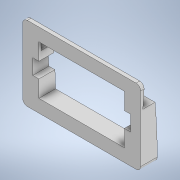
# Autodesk Inventor part: electricalCoverGasket02
Saved by Autodesk Inventor 2021.1 (Build 251245000, 245)
## iProperties
Created: 2020-08-29
Part Number: electricalCoverGasket02
Material: Generic
Document SubType Name: Modeling
Designer: robst
Density: 1 g/cm^3
Appearance: Default
Author: robst
Autodesk Inventor part; units mm, degrees
ref_plane "YZ Plane" through (0, 0, 0) normal (1, 0, 0) x (0, 1, 0)
ref_plane "XZ Plane" through (0, 0, 0) normal (0, 1, 0) x (-1, 0, 0)
sketch "Sketch1" plane through (0, 0, 0) normal (1, 0, 0) x (0, 1, 0)
  line L0 (0, 0) -> (0, 12.7)
  line L1 (0, 0) -> (-101.6, 0) construction
  arc A0 (-101.6, 0) -> (0, 0) centre (-50.8, 556.4861) ccw
  line L2 (-50.8, -2.3139) -> (-50.8, 0) construction
  line L3 (0, 12.7) -> (101.6, 12.7) construction
  arc A1 (0, 12.7) -> (101.6, 12.7) centre (50.8, 569.1861) ccw
  line L4 (22.2779, 14.9245) -> (-55.1921, 14.9245)
  line L5 (-55.1921, 14.9245) -> (-55.1921, -2.2966)
  line L6 (22.2779, 14.9245) -> (22.2779, 11.1145)
  dimension "d5" = 558.8
  dimension "d6" = 101.6
  dimension "d7" = 558.8
  dimension "d24" = 12.7
  dimension "d26" = 77.47
  dimension "d28" = 55.1921
  dimension "d29" = 3.81
  constraints: 14 end point, 7 point on circle, 3 horizontal, 2 centre point, 2 perpendicular, 1 midpoint, 1 vertical
  measures "d5" radius of A0
  measures "d6" distance of L0.end L3.end
  measures "d7" radius of A1
  measures "d24" distance of L0.start L0.end
  measures "d26" distance of L4.start L4.end
  measures "d28" distance between parallel lines of L0 L5
  measures "d29" distance of L4.start L6.end
extrude "Extrusion3" add sketch "Sketch1" along normal mid plane 122.428
sketch "Sketch5" plane through (0, 0, 0) normal (0, 0, 1) x (1, 0, 0)
  line L0 (-61.214, 22.2779) -> (61.214, 22.2779) projected
  line L1 (-61.214, 0) -> (61.214, 0) projected
  line L2 (61.214, 0) -> (61.214, 22.2779)
  line L3 (-61.214, 22.2779) -> (-61.214, 0)
  line L4 (61.214, 14.6579) -> (-61.214, 14.6579) construction
  line L5 (-61.214, -55.1921) -> (-61.214, 22.2779) construction
  line L6 (21.5694, 10.8479) -> (21.5694, 17.5664)
  line L7 (21.5694, 17.5664) -> (24.1259, 17.5664)
  line L8 (24.1259, 17.5664) -> (24.1259, 18.4679)
  line L9 (24.1259, 18.4679) -> (18.0002, 18.4679)
  line L10 (18.0002, 18.4679) -> (18.0002, 17.5664)
  line L11 (18.0002, 17.5664) -> (20.5567, 17.5664)
  line L12 (20.5567, 17.5664) -> (20.5567, 10.8479)
  line L13 (20.5567, 10.8479) -> (21.5694, 10.8479)
  spline S0 degree 2 poles (11.8314, 17.5972) (11.3991, 17.0909) (10.9175, 15.6089) (10.9175, 14.6579) knots 0 0 0 1 2 2 2
  spline S1 degree 2 poles (10.9175, 14.6579) (10.9175, 13.7317) (11.3868, 12.2311) (11.8314, 11.7248) knots 0 0 0 1 2 2 2
  spline S2 degree 2 poles (11.8314, 11.7248) (12.3007, 11.1937) (13.5419, 10.6874) (14.289, 10.6874) knots 0 0 0 1 2 2 2
  spline S3 degree 2 poles (14.289, 10.6874) (15.0609, 10.6874) (16.2959, 11.2122) (16.7467, 11.7248) knots 0 0 0 1 2 2 2
  spline S4 degree 2 poles (16.7467, 11.7248) (17.1851, 12.2311) (17.6544, 13.7193) (17.6544, 14.6579) knots 0 0 0 1 2 2 2
  spline S5 degree 2 poles (17.6544, 14.6579) (17.6544, 15.615) (17.179, 17.0724) (16.7405, 17.5972) knots 0 0 0 1 2 2 2
  spline S6 degree 2 poles (16.7405, 17.5972) (16.2959, 18.1036) (15.0547, 18.6285) (14.289, 18.6285) knots 0 0 0 1 2 2 2
  spline S7 degree 2 poles (14.289, 18.6285) (13.511, 18.6285) (12.2636, 18.0851) (11.8314, 17.5972) knots 0 0 0 1 2 2 2
  spline S8 degree 2 poles (11.9734, 14.6579) (11.9734, 15.4113) (12.3007, 16.5784) (12.5971, 16.9612) knots 0 0 0 1 2 2 2
  spline S9 degree 2 poles (12.5971, 16.9612) (12.8997, 17.3564) (13.7518, 17.7516) (14.2829, 17.7516) knots 0 0 0 1 2 2 2
  spline S10 degree 2 poles (14.2829, 17.7516) (14.8324, 17.7516) (15.6599, 17.3688) (15.9748, 16.9612) knots 0 0 0 1 2 2 2
  spline S11 degree 2 poles (15.9748, 16.9612) (16.2774, 16.5722) (16.5985, 15.3989) (16.5985, 14.6579) knots 0 0 0 1 2 2 2
  spline S12 degree 2 poles (16.5985, 14.6579) (16.5985, 13.1574) (15.3388, 11.5642) (14.2829, 11.5642) knots 0 0 0 1 2 2 2
  spline S13 degree 2 poles (14.2829, 11.5642) (13.2269, 11.5642) (11.9734, 13.1574) (11.9734, 14.6579) knots 0 0 0 1 2 2 2
  spline S14 degree 2 poles (4.9894, 16.1708) (4.9894, 15.6768) (5.3414, 14.7876) (5.6563, 14.4788) knots 0 0 0 1 2 2 2
  spline S15 degree 2 poles (5.6563, 14.4788) (6.0515, 14.0898) (7.1198, 13.6884) (7.9349, 13.6884) knots 0 0 0 1 2 2 2
  line L14 (7.9349, 13.6884) -> (8.7933, 13.6884)
  line L15 (8.7933, 13.6884) -> (8.7933, 10.8479)
  line L16 (8.7933, 10.8479) -> (9.806, 10.8479)
  line L17 (9.806, 10.8479) -> (9.806, 18.4679)
  line L18 (9.806, 18.4679) -> (7.8917, 18.4679)
  spline S16 degree 2 poles (7.8917, 18.4679) (7.2124, 18.4679) (6.2615, 18.2456) (5.8972, 17.9924) knots 0 0 0 1 2 2 2
  spline S17 degree 2 poles (5.8972, 17.9924) (5.4711, 17.7022) (4.9894, 16.8068) (4.9894, 16.1708) knots 0 0 0 1 2 2 2
  spline S18 degree 2 poles (6.0454, 16.1399) (6.0454, 16.5351) (6.3171, 17.1156) (6.5949, 17.3008) knots 0 0 0 1 2 2 2
  spline S19 degree 2 poles (6.5949, 17.3008) (6.8358, 17.4614) (7.478, 17.5911) (7.9535, 17.5911) knots 0 0 0 1 2 2 2
  line L19 (7.9535, 17.5911) -> (8.7933, 17.5911)
  line L20 (8.7933, 17.5911) -> (8.7933, 14.5529)
  line L21 (8.7933, 14.5529) -> (8.1017, 14.5529)
  spline S20 degree 2 poles (8.1017, 14.5529) (7.4841, 14.5529) (6.7246, 14.7505) (6.4776, 15.0099) knots 0 0 0 1 2 2 2
  spline S21 degree 2 poles (6.4776, 15.0099) (6.2491, 15.2384) (6.0454, 15.7756) (6.0454, 16.1399) knots 0 0 0 1 2 2 2
  line L22 (1.0745, 18.8075) -> (4.057, 9.193)
  line L23 (4.057, 9.193) -> (4.9215, 9.193)
  line L24 (4.9215, 9.193) -> (1.9513, 18.8075)
  line L25 (1.9513, 18.8075) -> (1.0745, 18.8075)
  spline S22 degree 2 poles (-5.15, 13.1883) (-5.15, 12.6202) (-4.7177, 11.7495) (-4.3596, 11.4654) knots 0 0 0 1 2 2 2
  spline S23 degree 2 poles (-4.3596, 11.4654) (-3.9273, 11.132) (-2.9455, 10.8479) (-2.1674, 10.8479) knots 0 0 0 1 2 2 2
  line L26 (-2.1674, 10.8479) -> (0.0185, 10.8479)
  line L27 (0.0185, 10.8479) -> (0.0185, 18.4679)
  line L28 (0.0185, 18.4679) -> (-2.0007, 18.4679)
  spline S24 degree 2 poles (-2.0007, 18.4679) (-2.8158, 18.4679) (-3.6309, 18.3629) (-4.0014, 18.1592) knots 0 0 0 1 2 2 2
  spline S25 degree 2 poles (-4.0014, 18.1592) (-4.4152, 17.943) (-4.7918, 17.2329) (-4.7918, 16.7513) knots 0 0 0 1 2 2 2
  spline S26 degree 2 poles (-4.7918, 16.7513) (-4.7918, 16.214) (-4.2237, 15.3619) (-3.7235, 15.121) knots 0 0 0 1 2 2 2
  line L29 (-3.7235, 15.121) -> (-3.7235, 15.084)
  spline S27 degree 2 poles (-3.7235, 15.084) (-4.4028, 14.8987) (-5.15, 13.9169) (-5.15, 13.1883) knots 0 0 0 1 2 2 2
  spline S28 degree 2 poles (-4.0941, 13.145) (-4.0941, 13.5773) (-3.8471, 14.133) (-3.4765, 14.3306) knots 0 0 0 1 2 2 2
  spline S29 degree 2 poles (-3.4765, 14.3306) (-3.2357, 14.4541) (-2.6676, 14.5282) (-2.1427, 14.5282) knots 0 0 0 1 2 2 2
  line L30 (-2.1427, 14.5282) -> (-0.9942, 14.5282)
  line L31 (-0.9942, 14.5282) -> (-0.9942, 11.7124)
  line L32 (-0.9942, 11.7124) -> (-1.8155, 11.7124)
  spline S30 degree 2 poles (-1.8155, 11.7124) (-2.4824, 11.7124) (-3.2481, 11.8359) (-3.5445, 12.0335) knots 0 0 0 1 2 2 2
  spline S31 degree 2 poles (-3.5445, 12.0335) (-3.8285, 12.2373) (-4.0941, 12.7437) (-4.0941, 13.145) knots 0 0 0 1 2 2 2
  spline S32 degree 2 poles (-3.7359, 16.6092) (-3.7359, 16.8809) (-3.5506, 17.2885) (-3.3469, 17.4058) knots 0 0 0 1 2 2 2
  spline S33 degree 2 poles (-3.3469, 17.4058) (-3.0999, 17.5417) (-2.5009, 17.6034) (-1.9637, 17.6034) knots 0 0 0 1 2 2 2
  line L33 (-1.9637, 17.6034) -> (-0.9942, 17.6034)
  line L34 (-0.9942, 17.6034) -> (-0.9942, 15.3742)
  line L35 (-0.9942, 15.3742) -> (-2.1427, 15.3742)
  spline S34 degree 2 poles (-2.1427, 15.3742) (-2.6182, 15.3742) (-3.069, 15.473) (-3.3098, 15.6274) knots 0 0 0 1 2 2 2
  spline S35 degree 2 poles (-3.3098, 15.6274) (-3.5445, 15.7756) (-3.7359, 16.2511) (-3.7359, 16.6092) knots 0 0 0 1 2 2 2
  line L36 (-5.3352, 10.8479) -> (-7.9041, 18.4679)
  line L37 (-7.9041, 18.4679) -> (-9.1514, 18.4679)
  line L38 (-9.1514, 18.4679) -> (-11.7202, 10.8479)
  line L39 (-11.7202, 10.8479) -> (-10.6519, 10.8479)
  line L40 (-10.6519, 10.8479) -> (-9.9603, 12.9783)
  line L41 (-9.9603, 12.9783) -> (-7.0519, 12.9783)
  line L42 (-7.0519, 12.9783) -> (-6.3603, 10.8479)
  line L43 (-6.3603, 10.8479) -> (-5.3352, 10.8479)
  line L44 (-9.6825, 13.8428) -> (-8.503, 17.4305)
  line L45 (-8.503, 17.4305) -> (-7.3298, 13.8428)
  line L46 (-7.3298, 13.8428) -> (-9.6825, 13.8428)
  spline S36 degree 2 poles (-15.5179, 10.7121) (-14.7769, 10.7121) (-13.5233, 11.2122) (-13.0664, 11.7124) knots 0 0 0 1 2 2 2
  spline S37 degree 2 poles (-13.0664, 11.7124) (-12.6094, 12.2064) (-12.1093, 13.6884) (-12.1093, 14.6517) knots 0 0 0 1 2 2 2
  spline S38 degree 2 poles (-12.1093, 14.6517) (-12.1093, 15.6089) (-12.5971, 17.0291) (-13.0602, 17.554) knots 0 0 0 1 2 2 2
  spline S39 degree 2 poles (-13.0602, 17.554) (-13.5172, 18.0665) (-14.7645, 18.6038) (-15.5364, 18.6038) knots 0 0 0 1 2 2 2
  spline S40 degree 2 poles (-15.5364, 18.6038) (-15.9193, 18.6038) (-16.5923, 18.4926) (-16.8764, 18.4062) knots 0 0 0 1 2 2 2
  spline S41 degree 2 poles (-16.8764, 18.4062) (-17.1234, 18.3259) (-17.6359, 18.0974) (-17.8891, 17.9616) knots 0 0 0 1 2 2 2
  line L47 (-17.8891, 17.9616) -> (-17.8891, 16.7389)
  line L48 (-17.8891, 16.7389) -> (-17.8088, 16.7389)
  spline S42 degree 2 poles (-17.8088, 16.7389) (-17.673, 16.8624) (-17.2531, 17.2082) (-16.9505, 17.3749) knots 0 0 0 1 2 2 2
  spline S43 degree 2 poles (-16.9505, 17.3749) (-16.6603, 17.5355) (-15.9748, 17.7393) (-15.5302, 17.7393) knots 0 0 0 1 2 2 2
  spline S44 degree 2 poles (-15.5302, 17.7393) (-15.0424, 17.7393) (-14.1717, 17.3379) (-13.8444, 16.955) knots 0 0 0 1 2 2 2
  spline S45 degree 2 poles (-13.8444, 16.955) (-13.5233, 16.566) (-13.1652, 15.3866) (-13.1652, 14.6517) knots 0 0 0 1 2 2 2
  spline S46 degree 2 poles (-13.1652, 14.6517) (-13.1652, 13.8675) (-13.5419, 12.7375) (-13.8691, 12.3485) knots 0 0 0 1 2 2 2
  spline S47 degree 2 poles (-13.8691, 12.3485) (-14.1902, 11.9718) (-15.0486, 11.5889) (-15.5302, 11.5889) knots 0 0 0 1 2 2 2
  spline S48 degree 2 poles (-15.5302, 11.5889) (-15.9687, 11.5889) (-16.7158, 11.805) (-17.0061, 11.9656) knots 0 0 0 1 2 2 2
  spline S49 degree 2 poles (-17.0061, 11.9656) (-17.2839, 12.1262) (-17.6977, 12.4596) (-17.815, 12.5769) knots 0 0 0 1 2 2 2
  line L49 (-17.815, 12.5769) -> (-17.8891, 12.5769)
  line L50 (-17.8891, 12.5769) -> (-17.8891, 11.3666)
  spline S50 degree 2 poles (-17.8891, 11.3666) (-17.6359, 11.2493) (-17.1913, 11.0332) (-16.8764, 10.9344) knots 0 0 0 1 2 2 2
  spline S51 degree 2 poles (-16.8764, 10.9344) (-16.5429, 10.8232) (-15.9748, 10.7121) (-15.5179, 10.7121) knots 0 0 0 1 2 2 2
  line L51 (-24.3914, 10.8479) -> (-23.0761, 10.8479)
  line L52 (-23.0761, 10.8479) -> (-20.2912, 14.3924)
  line L53 (-20.2912, 14.3924) -> (-19.8466, 13.8922)
  line L54 (-19.8466, 13.8922) -> (-19.8466, 10.8479)
  line L55 (-19.8466, 10.8479) -> (-18.8339, 10.8479)
  line L56 (-18.8339, 10.8479) -> (-18.8339, 18.4679)
  line L57 (-18.8339, 18.4679) -> (-19.8466, 18.4679)
  line L58 (-19.8466, 18.4679) -> (-19.8466, 14.9667)
  line L59 (-19.8466, 14.9667) -> (-22.9712, 18.4679)
  line L60 (-22.9712, 18.4679) -> (-24.2062, 18.4679)
  line L61 (-24.2062, 18.4679) -> (-21.0507, 15.0655)
  line L62 (-21.0507, 15.0655) -> (-24.3914, 10.8479)
  point P0 (0, 0)
  dimension "d41" = 7.62
  constraints: 6 end point, 1 horizontal
  measures "d41" distance between parallel lines of L4 L0
emboss "Emboss3" sketch "Sketch5" operation cut depth 1.016 direction (0, 0, -1) wrap yes faces at (20.4047, 12.3689, 11.7092) contours L13 L12 L11 L10 L9 L8 L7 L6 | S7 S6 S5 S4 S3 S2 S1 S0 | S17 S16 L18 L17 L16 L15 L14 S15 S14 | L25 L24 L23 L22 | S27 L29 S26 S25 S24 L28 L27 L26 S23 S22 | L43 L42 L41 L40 L39 L38 L37 L36 | S51 S50 L50 L49 S49 S48 S47 S46 S45 S44 S43 S42 L48 L47 S41 S40 S39 S38 S37 S36 | L62 L61 L60 L59 L58 L57 L56 L55 L54 L53 L52 L51
ref_plane "Work Plane3" through (0, -50.8, -2.3139) normal (0, 0, 1) x (1, 0, 0)
sketch "Sketch8" plane through (-61.214, -55.1921, 14.9245) normal (0, 0, 1) x (1, 0, 0)
  line L0 (122.428, 55.1921) -> (0, 55.1921) projected
  line L1 (61.214, 55.1921) -> (61.214, 0) construction
  line L2 (0, 0) -> (122.428, 0) construction
  line L3 (16.764, 13.335) -> (105.664, 13.335)
  line L4 (105.664, 13.335) -> (105.664, 64.135)
  line L5 (105.664, 64.135) -> (16.764, 64.135)
  line L6 (16.764, 64.135) -> (16.764, 13.335)
  line L7 (16.764, 13.335) -> (105.664, 64.135) construction
  line L8 (105.664, 13.335) -> (16.764, 64.135) construction
  point P0 (61.214, 38.735)
  dimension "d36" = 50.8
  dimension "d37" = 88.9
  dimension "d38" = 13.335
  constraints: 14 end point, 3 midpoint, 2 parallel, 2 perpendicular, 1 point on line
  measures "d36" distance of L5.end L3.start
  measures "d37" distance between parallel lines of L4 L6
  measures "d38" distance between parallel lines of L2 L3
extrude "Extrusion4" cut sketch "Sketch8" against normal through all
sketch "Sketch9" plane through (0, -50.8, -2.3139) normal (0, 0, 1) x (1, 0, 0)
  line L0 (-61.214, -4.3921) -> (61.214, -4.3921) projected
  line L1 (-44.45, 8.9429) -> (44.45, 8.9429) projected
  line L2 (-44.45, 8.9429) -> (-44.45, 59.7429) construction
  line L3 (-44.45, 8.9429) -> (-44.45, -4.3921) construction
  line L4 (-61.214, -4.3921) -> (61.214, -4.3921) construction
  line L5 (44.45, 8.9429) -> (-44.45, 8.9429) construction
  line L6 (44.45, 8.9429) -> (44.45, -4.3921) construction
  line L7 (44.45, 2.2754) -> (-44.45, 2.2754) construction
  spline S0 degree 2 poles (45.3685, -2.3209) (46.9679, -2.3209) (48.7257, -0.527) (48.7257, 1.1299) knots 0 0 0 1 2 2 2
  spline S1 degree 2 poles (48.7257, 1.1299) (48.7257, 2.7581) (47.0183, 4.6888) (45.6423, 4.6888) knots 0 0 0 1 2 2 2
  spline S2 degree 2 poles (45.6423, 4.6888) (45.0227, 4.6888) (44.0646, 4.3286) (43.7116, 3.9468) knots 0 0 0 1 2 2 2
  spline S3 degree 2 poles (43.7116, 3.9468) (43.3514, 3.565) (42.9695, 2.4627) (42.9695, 1.6631) knots 0 0 0 1 2 2 2
  line L8 (42.9695, 1.6631) -> (42.9695, 1.0507)
  line L9 (42.9695, 1.0507) -> (47.5874, 1.0507)
  spline S4 degree 2 poles (47.5874, 1.0507) (47.5874, -0.1092) (46.4204, -1.3411) (45.3829, -1.3411) knots 0 0 0 1 2 2 2
  spline S5 degree 2 poles (45.3829, -1.3411) (45.0155, -1.3411) (44.3023, -1.1754) (44.0141, -1.0457) knots 0 0 0 1 2 2 2
  spline S6 degree 2 poles (44.0141, -1.0457) (43.7116, -0.9016) (43.2937, -0.6495) (43.1568, -0.5342) knots 0 0 0 1 2 2 2
  line L10 (43.1568, -0.5342) -> (43.092, -0.5342)
  line L11 (43.092, -0.5342) -> (43.092, -1.7589)
  spline S7 degree 2 poles (43.092, -1.7589) (43.2865, -1.8382) (43.8773, -2.0687) (44.1078, -2.1336) knots 0 0 0 1 2 2 2
  spline S8 degree 2 poles (44.1078, -2.1336) (44.432, -2.2272) (44.9651, -2.3209) (45.3685, -2.3209) knots 0 0 0 1 2 2 2
  spline S9 degree 2 poles (44.0646, 1.908) (44.079, 2.3619) (44.2663, 3.0247) (44.4464, 3.248) knots 0 0 0 1 2 2 2
  spline S10 degree 2 poles (44.4464, 3.248) (44.6409, 3.5001) (45.2533, 3.7667) (45.7071, 3.7667) knots 0 0 0 1 2 2 2
  spline S11 degree 2 poles (45.7071, 3.7667) (46.1538, 3.7667) (46.7806, 3.5001) (47.0399, 3.2408) knots 0 0 0 1 2 2 2
  spline S12 degree 2 poles (47.0399, 3.2408) (47.2921, 2.9742) (47.5514, 2.3331) (47.5874, 1.908) knots 0 0 0 1 2 2 2
  line L12 (47.5874, 1.908) -> (44.0646, 1.908)
  spline S13 degree 2 poles (38.2724, -2.3281) (39.1369, -2.3281) (40.5993, -1.7445) (41.1325, -1.161) knots 0 0 0 1 2 2 2
  spline S14 degree 2 poles (41.1325, -1.161) (41.6656, -0.5847) (42.2491, 1.1444) (42.2491, 2.2682) knots 0 0 0 1 2 2 2
  spline S15 degree 2 poles (42.2491, 2.2682) (42.2491, 3.3849) (41.68, 5.0418) (41.1397, 5.6542) knots 0 0 0 1 2 2 2
  spline S16 degree 2 poles (41.1397, 5.6542) (40.6066, 6.2521) (39.1513, 6.8789) (38.2508, 6.8789) knots 0 0 0 1 2 2 2
  spline S17 degree 2 poles (38.2508, 6.8789) (37.8041, 6.8789) (37.0189, 6.7492) (36.6875, 6.6484) knots 0 0 0 1 2 2 2
  spline S18 degree 2 poles (36.6875, 6.6484) (36.3993, 6.5547) (35.8013, 6.2882) (35.506, 6.1297) knots 0 0 0 1 2 2 2
  line L13 (35.506, 6.1297) -> (35.506, 4.7032)
  line L14 (35.506, 4.7032) -> (35.5996, 4.7032)
  spline S19 degree 2 poles (35.5996, 4.7032) (35.7581, 4.8473) (36.248, 5.2508) (36.601, 5.4453) knots 0 0 0 1 2 2 2
  spline S20 degree 2 poles (36.601, 5.4453) (36.9396, 5.6326) (37.7393, 5.8703) (38.258, 5.8703) knots 0 0 0 1 2 2 2
  spline S21 degree 2 poles (38.258, 5.8703) (38.8271, 5.8703) (39.8429, 5.402) (40.2247, 4.9554) knots 0 0 0 1 2 2 2
  spline S22 degree 2 poles (40.2247, 4.9554) (40.5993, 4.5015) (41.0172, 3.1255) (41.0172, 2.2682) knots 0 0 0 1 2 2 2
  spline S23 degree 2 poles (41.0172, 2.2682) (41.0172, 1.3533) (40.5777, 0.0349) (40.1959, -0.419) knots 0 0 0 1 2 2 2
  spline S24 degree 2 poles (40.1959, -0.419) (39.8213, -0.8584) (38.8199, -1.3051) (38.258, -1.3051) knots 0 0 0 1 2 2 2
  spline S25 degree 2 poles (38.258, -1.3051) (37.7465, -1.3051) (36.8748, -1.0529) (36.5362, -0.8656) knots 0 0 0 1 2 2 2
  spline S26 degree 2 poles (36.5362, -0.8656) (36.212, -0.6783) (35.7293, -0.2893) (35.5924, -0.1524) knots 0 0 0 1 2 2 2
  line L15 (35.5924, -0.1524) -> (35.506, -0.1524)
  line L16 (35.506, -0.1524) -> (35.506, -1.5644)
  spline S27 degree 2 poles (35.506, -1.5644) (35.8013, -1.7013) (36.32, -1.9535) (36.6875, -2.0687) knots 0 0 0 1 2 2 2
  spline S28 degree 2 poles (36.6875, -2.0687) (37.0765, -2.1984) (37.7393, -2.3281) (38.2724, -2.3281) knots 0 0 0 1 2 2 2
  spline S29 degree 2 poles (30.6791, -2.3425) (31.6229, -2.3425) (33.1862, -1.7661) (33.7481, -1.1826) knots 0 0 0 1 2 2 2
  spline S30 degree 2 poles (33.7481, -1.1826) (34.3101, -0.5919) (34.908, 1.1516) (34.908, 2.2826) knots 0 0 0 1 2 2 2
  spline S31 degree 2 poles (34.908, 2.2826) (34.908, 3.356) (34.3029, 5.0562) (33.7409, 5.6614) knots 0 0 0 1 2 2 2
  spline S32 degree 2 poles (33.7409, 5.6614) (33.2006, 6.2449) (31.6157, 6.8789) (30.6719, 6.8789) knots 0 0 0 1 2 2 2
  spline S33 degree 2 poles (30.6719, 6.8789) (30.2181, 6.8789) (29.3968, 6.7492) (29.0222, 6.634) knots 0 0 0 1 2 2 2
  spline S34 degree 2 poles (29.0222, 6.634) (28.7196, 6.5475) (27.9848, 6.2305) (27.7614, 6.1153) knots 0 0 0 1 2 2 2
  line L17 (27.7614, 6.1153) -> (27.7614, 4.6888)
  line L18 (27.7614, 4.6888) -> (27.8623, 4.6888)
  spline S35 degree 2 poles (27.8623, 4.6888) (28.0856, 4.8833) (28.5539, 5.2363) (28.9862, 5.4381) knots 0 0 0 1 2 2 2
  spline S36 degree 2 poles (28.9862, 5.4381) (29.3464, 5.6182) (30.2757, 5.8559) (30.8088, 5.8559) knots 0 0 0 1 2 2 2
  spline S37 degree 2 poles (30.8088, 5.8559) (32.0912, 5.8559) (33.6761, 3.9252) (33.6761, 2.3186) knots 0 0 0 1 2 2 2
  spline S38 degree 2 poles (33.6761, 2.3186) (33.6761, 1.4253) (33.2583, 0.0853) (32.862, -0.3757) knots 0 0 0 1 2 2 2
  spline S39 degree 2 poles (32.862, -0.3757) (32.4802, -0.8368) (31.3996, -1.3195) (30.7224, -1.3195) knots 0 0 0 1 2 2 2
  spline S40 degree 2 poles (30.7224, -1.3195) (30.2253, -1.3195) (29.2311, -1.1754) (28.8925, -1.0313) knots 0 0 0 1 2 2 2
  line L19 (28.8925, -1.0313) -> (28.8925, 1.2668)
  line L20 (28.8925, 1.2668) -> (30.9529, 1.2668)
  line L21 (30.9529, 1.2668) -> (30.9529, 2.3042)
  line L22 (30.9529, 2.3042) -> (27.7254, 2.3042)
  line L23 (27.7254, 2.3042) -> (27.7254, -1.5788)
  spline S41 degree 2 poles (27.7254, -1.5788) (27.9487, -1.6797) (28.7124, -1.9895) (29.0366, -2.0831) knots 0 0 0 1 2 2 2
  spline S42 degree 2 poles (29.0366, -2.0831) (29.476, -2.2128) (30.1821, -2.3425) (30.6791, -2.3425) knots 0 0 0 1 2 2 2
  spline S43 degree 2 poles (20.9607, 2.2754) (20.9607, -0.1164) (22.3511, -2.3569) (23.7991, -2.3569) knots 0 0 0 1 2 2 2
  spline S44 degree 2 poles (23.7991, -2.3569) (25.2688, -2.3569) (26.6448, -0.0732) (26.6448, 2.2682) knots 0 0 0 1 2 2 2
  spline S45 degree 2 poles (26.6448, 2.2682) (26.6448, 4.6744) (25.2544, 6.9005) (23.7991, 6.9005) knots 0 0 0 1 2 2 2
  spline S46 degree 2 poles (23.7991, 6.9005) (22.3367, 6.9005) (20.9607, 4.5952) (20.9607, 2.2754) knots 0 0 0 1 2 2 2
  spline S47 degree 2 poles (22.488, -0.4334) (22.3151, 0.0061) (22.171, 1.3605) (22.171, 2.2754) knots 0 0 0 1 2 2 2
  spline S48 degree 2 poles (22.171, 2.2754) (22.171, 3.1904) (22.3151, 4.5375) (22.4952, 4.9914) knots 0 0 0 1 2 2 2
  spline S49 degree 2 poles (22.4952, 4.9914) (22.6753, 5.4453) (23.302, 5.9135) (23.7991, 5.9135) knots 0 0 0 1 2 2 2
  spline S50 degree 2 poles (23.7991, 5.9135) (24.2962, 5.9135) (24.9374, 5.4453) (25.1247, 4.977) knots 0 0 0 1 2 2 2
  spline S51 degree 2 poles (25.1247, 4.977) (25.3048, 4.5231) (25.4345, 3.1399) (25.4345, 2.2682) knots 0 0 0 1 2 2 2
  spline S52 degree 2 poles (25.4345, 2.2682) (25.4345, 1.3317) (25.3192, 0.0781) (25.1319, -0.4118) knots 0 0 0 1 2 2 2
  spline S53 degree 2 poles (25.1319, -0.4118) (24.959, -0.8728) (24.3178, -1.3699) (23.7991, -1.3699) knots 0 0 0 1 2 2 2
  spline S54 degree 2 poles (23.7991, -1.3699) (23.3092, -1.3699) (22.6681, -0.9016) (22.488, -0.4334) knots 0 0 0 1 2 2 2
  line L24 (14.34, -2.1696) -> (19.8224, -2.1696)
  line L25 (19.8224, -2.1696) -> (19.8224, -0.9088)
  spline S55 degree 2 poles (19.8224, -0.9088) (19.2316, -0.3541) (18.1798, 0.6761) (17.6755, 1.2308) knots 0 0 0 1 2 2 2
  spline S56 degree 2 poles (17.6755, 1.2308) (16.6597, 2.3475) (15.9177, 3.6874) (15.9177, 4.4007) knots 0 0 0 1 2 2 2
  spline S57 degree 2 poles (15.9177, 4.4007) (15.9177, 4.7753) (16.1482, 5.3372) (16.3572, 5.5173) knots 0 0 0 1 2 2 2
  spline S58 degree 2 poles (16.3572, 5.5173) (16.5661, 5.6974) (17.1136, 5.8775) (17.445, 5.8775) knots 0 0 0 1 2 2 2
  spline S59 degree 2 poles (17.445, 5.8775) (17.762, 5.8775) (18.4104, 5.719) (18.7057, 5.5966) knots 0 0 0 1 2 2 2
  spline S60 degree 2 poles (18.7057, 5.5966) (18.9579, 5.4957) (19.4262, 5.2075) (19.5702, 5.1067) knots 0 0 0 1 2 2 2
  line L26 (19.5702, 5.1067) -> (19.6351, 5.1067)
  line L27 (19.6351, 5.1067) -> (19.6351, 6.3746)
  spline S61 degree 2 poles (19.6351, 6.3746) (19.2677, 6.5547) (17.9493, 6.9077) (17.3586, 6.9077) knots 0 0 0 1 2 2 2
  spline S62 degree 2 poles (17.3586, 6.9077) (16.1122, 6.9077) (14.7074, 5.5894) (14.7074, 4.4655) knots 0 0 0 1 2 2 2
  spline S63 degree 2 poles (14.7074, 4.4655) (14.7074, 3.9396) (14.9523, 3.0607) (15.1685, 2.6861) knots 0 0 0 1 2 2 2
  spline S64 degree 2 poles (15.1685, 2.6861) (15.3846, 2.297) (16.0114, 1.5334) (16.3572, 1.166) knots 0 0 0 1 2 2 2
  spline S65 degree 2 poles (16.3572, 1.166) (16.9191, 0.5536) (18.2951, -0.7576) (18.7057, -1.1394) knots 0 0 0 1 2 2 2
  line L28 (18.7057, -1.1394) -> (14.34, -1.1394)
  line L29 (14.34, -1.1394) -> (14.34, -2.1696)
  spline S66 degree 2 poles (3.4616, 4.0404) (3.4616, 3.4641) (3.8723, 2.4267) (4.2397, 2.0665) knots 0 0 0 1 2 2 2
  spline S67 degree 2 poles (4.2397, 2.0665) (4.7008, 1.6126) (5.9471, 1.1444) (6.898, 1.1444) knots 0 0 0 1 2 2 2
  line L30 (6.898, 1.1444) -> (7.8994, 1.1444)
  line L31 (7.8994, 1.1444) -> (7.8994, -2.1696)
  line L32 (7.8994, -2.1696) -> (9.0809, -2.1696)
  line L33 (9.0809, -2.1696) -> (9.0809, 6.7204)
  line L34 (9.0809, 6.7204) -> (6.8476, 6.7204)
  spline S68 degree 2 poles (6.8476, 6.7204) (6.0551, 6.7204) (4.9457, 6.4611) (4.5206, 6.1657) knots 0 0 0 1 2 2 2
  spline S69 degree 2 poles (4.5206, 6.1657) (4.0236, 5.8271) (3.4616, 4.7825) (3.4616, 4.0404) knots 0 0 0 1 2 2 2
  spline S70 degree 2 poles (4.6935, 4.0044) (4.6935, 4.4655) (5.0105, 5.1427) (5.3347, 5.3588) knots 0 0 0 1 2 2 2
  spline S71 degree 2 poles (5.3347, 5.3588) (5.6157, 5.5461) (6.3649, 5.6974) (6.9196, 5.6974) knots 0 0 0 1 2 2 2
  line L35 (6.9196, 5.6974) -> (7.8994, 5.6974)
  line L36 (7.8994, 5.6974) -> (7.8994, 2.1529)
  line L37 (7.8994, 2.1529) -> (7.0925, 2.1529)
  spline S72 degree 2 poles (7.0925, 2.1529) (6.3721, 2.1529) (5.486, 2.3835) (5.1978, 2.6861) knots 0 0 0 1 2 2 2
  spline S73 degree 2 poles (5.1978, 2.6861) (4.9313, 2.9526) (4.6935, 3.5794) (4.6935, 4.0044) knots 0 0 0 1 2 2 2
  line L38 (-2.8132, 4.5015) -> (-0.299, -2.1696)
  line L39 (-0.299, -2.1696) -> (0.7096, -2.1696)
  line L40 (0.7096, -2.1696) -> (3.2023, 4.5015)
  line L41 (3.2023, 4.5015) -> (1.9848, 4.5015)
  line L42 (1.9848, 4.5015) -> (0.1621, -0.6351)
  line L43 (0.1621, -0.6351) -> (-1.6462, 4.5015)
  line L44 (-1.6462, 4.5015) -> (-2.8132, 4.5015)
  spline S74 degree 2 poles (-9.0305, 2.2754) (-9.0305, -0.1164) (-7.6401, -2.3569) (-6.192, -2.3569) knots 0 0 0 1 2 2 2
  spline S75 degree 2 poles (-6.192, -2.3569) (-4.7224, -2.3569) (-3.3464, -0.0732) (-3.3464, 2.2682) knots 0 0 0 1 2 2 2
  spline S76 degree 2 poles (-3.3464, 2.2682) (-3.3464, 4.6744) (-4.7368, 6.9005) (-6.192, 6.9005) knots 0 0 0 1 2 2 2
  spline S77 degree 2 poles (-6.192, 6.9005) (-7.6545, 6.9005) (-9.0305, 4.5952) (-9.0305, 2.2754) knots 0 0 0 1 2 2 2
  spline S78 degree 2 poles (-7.5032, -0.4334) (-7.6761, 0.0061) (-7.8202, 1.3605) (-7.8202, 2.2754) knots 0 0 0 1 2 2 2
  spline S79 degree 2 poles (-7.8202, 2.2754) (-7.8202, 3.1904) (-7.6761, 4.5375) (-7.496, 4.9914) knots 0 0 0 1 2 2 2
  spline S80 degree 2 poles (-7.496, 4.9914) (-7.3159, 5.4453) (-6.6891, 5.9135) (-6.192, 5.9135) knots 0 0 0 1 2 2 2
  spline S81 degree 2 poles (-6.192, 5.9135) (-5.6949, 5.9135) (-5.0538, 5.4453) (-4.8664, 4.977) knots 0 0 0 1 2 2 2
  spline S82 degree 2 poles (-4.8664, 4.977) (-4.6863, 4.5231) (-4.5567, 3.1399) (-4.5567, 2.2682) knots 0 0 0 1 2 2 2
  spline S83 degree 2 poles (-4.5567, 2.2682) (-4.5567, 1.3317) (-4.6719, 0.0781) (-4.8592, -0.4118) knots 0 0 0 1 2 2 2
  spline S84 degree 2 poles (-4.8592, -0.4118) (-5.0321, -0.8728) (-5.6733, -1.3699) (-6.192, -1.3699) knots 0 0 0 1 2 2 2
  spline S85 degree 2 poles (-6.192, -1.3699) (-6.6819, -1.3699) (-7.3231, -0.9016) (-7.5032, -0.4334) knots 0 0 0 1 2 2 2
  line L45 (-15.6512, -2.1696) -> (-10.1687, -2.1696)
  line L46 (-10.1687, -2.1696) -> (-10.1687, -0.9088)
  spline S86 degree 2 poles (-10.1687, -0.9088) (-10.7595, -0.3541) (-11.8113, 0.6761) (-12.3156, 1.2308) knots 0 0 0 1 2 2 2
  spline S87 degree 2 poles (-12.3156, 1.2308) (-13.3314, 2.3475) (-14.0734, 3.6874) (-14.0734, 4.4007) knots 0 0 0 1 2 2 2
  spline S88 degree 2 poles (-14.0734, 4.4007) (-14.0734, 4.7753) (-13.8429, 5.3372) (-13.634, 5.5173) knots 0 0 0 1 2 2 2
  spline S89 degree 2 poles (-13.634, 5.5173) (-13.4251, 5.6974) (-12.8775, 5.8775) (-12.5461, 5.8775) knots 0 0 0 1 2 2 2
  spline S90 degree 2 poles (-12.5461, 5.8775) (-12.2292, 5.8775) (-11.5808, 5.719) (-11.2854, 5.5966) knots 0 0 0 1 2 2 2
  spline S91 degree 2 poles (-11.2854, 5.5966) (-11.0333, 5.4957) (-10.565, 5.2075) (-10.4209, 5.1067) knots 0 0 0 1 2 2 2
  line L47 (-10.4209, 5.1067) -> (-10.3561, 5.1067)
  line L48 (-10.3561, 5.1067) -> (-10.3561, 6.3746)
  spline S92 degree 2 poles (-10.3561, 6.3746) (-10.7235, 6.5547) (-12.0418, 6.9077) (-12.6326, 6.9077) knots 0 0 0 1 2 2 2
  spline S93 degree 2 poles (-12.6326, 6.9077) (-13.8789, 6.9077) (-15.2837, 5.5894) (-15.2837, 4.4655) knots 0 0 0 1 2 2 2
  spline S94 degree 2 poles (-15.2837, 4.4655) (-15.2837, 3.9396) (-15.0388, 3.0607) (-14.8227, 2.6861) knots 0 0 0 1 2 2 2
  spline S95 degree 2 poles (-14.8227, 2.6861) (-14.6065, 2.297) (-13.9798, 1.5334) (-13.634, 1.166) knots 0 0 0 1 2 2 2
  spline S96 degree 2 poles (-13.634, 1.166) (-13.072, 0.5536) (-11.696, -0.7576) (-11.2854, -1.1394) knots 0 0 0 1 2 2 2
  line L49 (-11.2854, -1.1394) -> (-15.6512, -1.1394)
  line L50 (-15.6512, -1.1394) -> (-15.6512, -2.1696)
  spline S97 degree 2 poles (-26.9402, 0.5608) (-26.9402, -0.102) (-26.4359, -1.1178) (-26.018, -1.4492) knots 0 0 0 1 2 2 2
  spline S98 degree 2 poles (-26.018, -1.4492) (-25.5137, -1.8382) (-24.3683, -2.1696) (-23.4605, -2.1696) knots 0 0 0 1 2 2 2
  line L51 (-23.4605, -2.1696) -> (-20.9102, -2.1696)
  line L52 (-20.9102, -2.1696) -> (-20.9102, 6.7204)
  line L53 (-20.9102, 6.7204) -> (-23.266, 6.7204)
  spline S99 degree 2 poles (-23.266, 6.7204) (-24.217, 6.7204) (-25.1679, 6.5979) (-25.6002, 6.3602) knots 0 0 0 1 2 2 2
  spline S100 degree 2 poles (-25.6002, 6.3602) (-26.0829, 6.1081) (-26.5223, 5.2796) (-26.5223, 4.7176) knots 0 0 0 1 2 2 2
  spline S101 degree 2 poles (-26.5223, 4.7176) (-26.5223, 4.0909) (-25.8595, 3.0967) (-25.276, 2.8157) knots 0 0 0 1 2 2 2
  line L54 (-25.276, 2.8157) -> (-25.276, 2.7725)
  spline S102 degree 2 poles (-25.276, 2.7725) (-26.0684, 2.5564) (-26.9402, 1.4109) (-26.9402, 0.5608) knots 0 0 0 1 2 2 2
  spline S103 degree 2 poles (-25.7082, 0.5104) (-25.7082, 1.0147) (-25.4201, 1.6631) (-24.9878, 1.8936) knots 0 0 0 1 2 2 2
  spline S104 degree 2 poles (-24.9878, 1.8936) (-24.7068, 2.0377) (-24.0441, 2.1241) (-23.4317, 2.1241) knots 0 0 0 1 2 2 2
  line L55 (-23.4317, 2.1241) -> (-22.0917, 2.1241)
  line L56 (-22.0917, 2.1241) -> (-22.0917, -1.161)
  line L57 (-22.0917, -1.161) -> (-23.0499, -1.161)
  spline S105 degree 2 poles (-23.0499, -1.161) (-23.8279, -1.161) (-24.7213, -1.0169) (-25.0671, -0.7864) knots 0 0 0 1 2 2 2
  spline S106 degree 2 poles (-25.0671, -0.7864) (-25.3985, -0.5486) (-25.7082, 0.0421) (-25.7082, 0.5104) knots 0 0 0 1 2 2 2
  spline S107 degree 2 poles (-25.2904, 4.5519) (-25.2904, 4.8689) (-25.0743, 5.3444) (-24.8365, 5.4813) knots 0 0 0 1 2 2 2
  spline S108 degree 2 poles (-24.8365, 5.4813) (-24.5484, 5.6398) (-23.8495, 5.7118) (-23.2228, 5.7118) knots 0 0 0 1 2 2 2
  line L58 (-23.2228, 5.7118) -> (-22.0917, 5.7118)
  line L59 (-22.0917, 5.7118) -> (-22.0917, 3.1111)
  line L60 (-22.0917, 3.1111) -> (-23.4317, 3.1111)
  spline S109 degree 2 poles (-23.4317, 3.1111) (-23.9864, 3.1111) (-24.5123, 3.2264) (-24.7933, 3.4065) knots 0 0 0 1 2 2 2
  spline S110 degree 2 poles (-24.7933, 3.4065) (-25.0671, 3.5794) (-25.2904, 4.1341) (-25.2904, 4.5519) knots 0 0 0 1 2 2 2
  line L61 (-27.1563, -2.1696) -> (-30.1532, 6.7204)
  line L62 (-30.1532, 6.7204) -> (-31.6085, 6.7204)
  line L63 (-31.6085, 6.7204) -> (-34.6054, -2.1696)
  line L64 (-34.6054, -2.1696) -> (-33.3591, -2.1696)
  line L65 (-33.3591, -2.1696) -> (-32.5522, 0.3159)
  line L66 (-32.5522, 0.3159) -> (-29.1591, 0.3159)
  line L67 (-29.1591, 0.3159) -> (-28.3522, -2.1696)
  line L68 (-28.3522, -2.1696) -> (-27.1563, -2.1696)
  line L69 (-32.228, 1.3245) -> (-30.852, 5.5101)
  line L70 (-30.852, 5.5101) -> (-29.4832, 1.3245)
  line L71 (-29.4832, 1.3245) -> (-32.228, 1.3245)
  spline S111 degree 2 poles (-39.036, -2.3281) (-38.1715, -2.3281) (-36.7091, -1.7445) (-36.176, -1.161) knots 0 0 0 1 2 2 2
  spline S112 degree 2 poles (-36.176, -1.161) (-35.6428, -0.5847) (-35.0593, 1.1444) (-35.0593, 2.2682) knots 0 0 0 1 2 2 2
  spline S113 degree 2 poles (-35.0593, 2.2682) (-35.0593, 3.3849) (-35.6284, 5.0418) (-36.1688, 5.6542) knots 0 0 0 1 2 2 2
  spline S114 degree 2 poles (-36.1688, 5.6542) (-36.7019, 6.2521) (-38.1571, 6.8789) (-39.0576, 6.8789) knots 0 0 0 1 2 2 2
  spline S115 degree 2 poles (-39.0576, 6.8789) (-39.5043, 6.8789) (-40.2896, 6.7492) (-40.621, 6.6484) knots 0 0 0 1 2 2 2
  spline S116 degree 2 poles (-40.621, 6.6484) (-40.9091, 6.5547) (-41.5071, 6.2882) (-41.8024, 6.1297) knots 0 0 0 1 2 2 2
  line L72 (-41.8024, 6.1297) -> (-41.8024, 4.7032)
  line L73 (-41.8024, 4.7032) -> (-41.7088, 4.7032)
  spline S117 degree 2 poles (-41.7088, 4.7032) (-41.5503, 4.8473) (-41.0604, 5.2508) (-40.7074, 5.4453) knots 0 0 0 1 2 2 2
  spline S118 degree 2 poles (-40.7074, 5.4453) (-40.3688, 5.6326) (-39.5691, 5.8703) (-39.0504, 5.8703) knots 0 0 0 1 2 2 2
  spline S119 degree 2 poles (-39.0504, 5.8703) (-38.4813, 5.8703) (-37.4655, 5.402) (-37.0837, 4.9554) knots 0 0 0 1 2 2 2
  spline S120 degree 2 poles (-37.0837, 4.9554) (-36.7091, 4.5015) (-36.2912, 3.1255) (-36.2912, 2.2682) knots 0 0 0 1 2 2 2
  spline S121 degree 2 poles (-36.2912, 2.2682) (-36.2912, 1.3533) (-36.7307, 0.0349) (-37.1125, -0.419) knots 0 0 0 1 2 2 2
  spline S122 degree 2 poles (-37.1125, -0.419) (-37.4871, -0.8584) (-38.4885, -1.3051) (-39.0504, -1.3051) knots 0 0 0 1 2 2 2
  spline S123 degree 2 poles (-39.0504, -1.3051) (-39.5619, -1.3051) (-40.4336, -1.0529) (-40.7722, -0.8656) knots 0 0 0 1 2 2 2
  spline S124 degree 2 poles (-40.7722, -0.8656) (-41.0964, -0.6783) (-41.5791, -0.2893) (-41.716, -0.1524) knots 0 0 0 1 2 2 2
  line L74 (-41.716, -0.1524) -> (-41.8024, -0.1524)
  line L75 (-41.8024, -0.1524) -> (-41.8024, -1.5644)
  spline S125 degree 2 poles (-41.8024, -1.5644) (-41.5071, -1.7013) (-40.9884, -1.9535) (-40.621, -2.0687) knots 0 0 0 1 2 2 2
  spline S126 degree 2 poles (-40.621, -2.0687) (-40.2319, -2.1984) (-39.5691, -2.3281) (-39.036, -2.3281) knots 0 0 0 1 2 2 2
  line L76 (-49.3885, -2.1696) -> (-47.854, -2.1696)
  line L77 (-47.854, -2.1696) -> (-44.6049, 1.9656)
  line L78 (-44.6049, 1.9656) -> (-44.0862, 1.3821)
  line L79 (-44.0862, 1.3821) -> (-44.0862, -2.1696)
  line L80 (-44.0862, -2.1696) -> (-42.9047, -2.1696)
  line L81 (-42.9047, -2.1696) -> (-42.9047, 6.7204)
  line L82 (-42.9047, 6.7204) -> (-44.0862, 6.7204)
  line L83 (-44.0862, 6.7204) -> (-44.0862, 2.6356)
  line L84 (-44.0862, 2.6356) -> (-47.7315, 6.7204)
  line L85 (-47.7315, 6.7204) -> (-49.1724, 6.7204)
  line L86 (-49.1724, 6.7204) -> (-45.491, 2.7509)
  line L87 (-45.491, 2.7509) -> (-49.3885, -2.1696)
  point P0 (0, 50.8)
  constraints: 6 end point, 2 midpoint, 2 perpendicular, 2 point on line, 1 horizontal
emboss "Emboss5" sketch "Sketch9" operation cut depth 1.016 direction (0, 0, -1) wrap yes faces at (-14.8167, -50.747, -2.3139)
fillet "Fillet1" radius 4.7625 4 edges at (-61.214, 22.2779, 13.0195) (-61.214, -55.1921, 6.3139) (61.214, -55.1921, 6.3139) (61.214, 22.2779, 13.0195)
sketch "Sketch10" plane through (-56.4515, 22.2779, 14.9245) normal (0, 0, 1) x (1, 0, 0)
  line L0 (12.0015, -64.135) -> (12.0015, -13.335) projected
  line L1 (12.0015, -13.335) -> (100.9015, -13.335) projected
  line L2 (100.9015, -13.335) -> (100.9015, -64.135) projected
  line L3 (100.9015, -64.135) -> (12.0015, -64.135) projected
  line L4 (12.0015, -13.335) -> (12.0015, -22.2779) construction
  line L5 (12.0015, -38.735) -> (100.9015, -38.735) construction
  line L6 (5.6515, -46.6725) -> (18.3515, -46.6725)
  line L7 (18.3515, -46.6725) -> (18.3515, -30.7975)
  line L8 (18.3515, -30.7975) -> (5.6515, -30.7975)
  line L9 (5.6515, -30.7975) -> (5.6515, -46.6725)
  line L10 (5.6515, -46.6725) -> (18.3515, -30.7975) construction
  line L11 (18.3515, -46.6725) -> (5.6515, -30.7975) construction
  line L12 (94.5515, -46.6725) -> (107.2515, -46.6725)
  line L13 (107.2515, -46.6725) -> (107.2515, -30.7975)
  line L14 (107.2515, -30.7975) -> (94.5515, -30.7975)
  line L15 (94.5515, -30.7975) -> (94.5515, -46.6725)
  line L16 (94.5515, -46.6725) -> (107.2515, -30.7975) construction
  line L17 (107.2515, -46.6725) -> (94.5515, -30.7975) construction
  line L18 (100.9015, -64.135) -> (100.9015, -22.2779) projected
  point P0 (56.4515, -22.2779)
  point P1 (100.9015, -30.7975)
  point P2 (100.9015, -46.6725)
  point P3 (12.0015, -46.6725)
  point P4 (12.0015, -30.7975)
  dimension "d45" = 25.4
  dimension "d46" = 12.7
  dimension "d47" = 15.875
  constraints: 26 end point, 5 midpoint, 4 parallel, 4 perpendicular, 2 equal length, 1 point on line
  measures "d45" distance between parallel lines of L5 L1
  measures "d46" distance of L7.end L8.end
  measures "d47" distance of L8.end L6.start
extrude "Extrusion5" cut sketch "Sketch10" against normal through all contours L6 L9 L8 L0 | L2 L14 L13 L12
equation "\"d5\" = radiusOfCurvature"
equation "\"d6\" = sidingHeight"
equation "\"d7\" = radiusOfCurvature"
equation "\"d24\" = sidingDepth"
equation "\"d26\" = coverHeight"
equation "\"d29\" = partMinDepth"
equation "\"d30\" = coverWidth"
equation "\"d32\" = textDepth"
equation "\"d36\" = insideHoleHeight"
equation "\"d37\" = insideHoleWidth"
equation "\"d42\" = textDepth"
equation "\"d44\" = filletRadiusAroundEdges"
equation "\"d45\" = 0.5 * insideHoleHeight"
equation "\"sidingHeight\" = 101.6"
equation "\"sidingDepth\" = 12.7"
equation "\"radiusOfCurvature\" = 558.8"
equation "\"partMinDepth\" = 3.81"
equation "\"coverHeight\" = 77.47"
equation "\"coverWidth\" = 122.428"
equation "\"electricalPlugHeight\" = 38.1"
equation "\"insideHoleWidth\" = 88.9"
equation "\"insideHoleHeight\" = 50.8"
equation "\"textDepth\" = 1.016"
equation "\"textCenterLine\" = 6.6675"
equation "\"filletRadiusAroundEdges\" = 4.7625"
body "Solid1"
body "Solid2"
